Autodesk Inventor part; units mm, degrees
(part 2 of 4)
sketch "Sketch7" plane through (0, 0, 0.5) normal (0, 0, 1) x (1, 0, 0)
  line L0 (29.16, -27.5) -> (28.16, -27.5)
  line L1 (28.16, -27.5) -> (28.16, -25)
  line L2 (28.16, -25) -> (29.16, -25)
  line L3 (29.16, -25) -> (29.16, -27.5)
  line L4 (24.08, -27.5) -> (23.08, -27.5)
  line L5 (23.08, -27.5) -> (23.08, -25)
  line L6 (23.08, -25) -> (24.08, -25)
  line L7 (24.08, -25) -> (24.08, -27.5)
  line L8 (19, -25) -> (19, -27.5)
  line L9 (19, -27.5) -> (18, -27.5)
  line L10 (18, -27.5) -> (18, -25)
  line L11 (18, -25) -> (19, -25)
  line L12 (14.85, -3.9) -> (13.65, -3.9)
  line L13 (13.65, -3.9) -> (13.65, -3.6)
  line L14 (13.65, -3.6) -> (14.85, -3.6)
  line L15 (14.85, -3.6) -> (14.85, -3.9)
  line L16 (14.85, -3.4) -> (13.65, -3.4)
  line L17 (13.65, -3.4) -> (13.65, -3.1)
  line L18 (13.65, -3.1) -> (14.85, -3.1)
  line L19 (14.85, -3.1) -> (14.85, -3.4)
  line L20 (14.85, -2.9) -> (13.65, -2.9)
  line L21 (13.65, -2.9) -> (13.65, -2.6)
  line L22 (13.65, -2.6) -> (14.85, -2.6)
  line L23 (14.85, -2.6) -> (14.85, -2.9)
  line L24 (14.85, -2.4) -> (13.65, -2.4)
  line L25 (13.65, -2.4) -> (13.65, -2.1)
  line L26 (13.65, -2.1) -> (14.85, -2.1)
  line L27 (14.85, -2.1) -> (14.85, -2.4)
  line L28 (14.85, -1.9) -> (13.65, -1.9)
  line L29 (13.65, -1.9) -> (13.65, -1.6)
  line L30 (13.65, -1.6) -> (14.85, -1.6)
  line L31 (14.85, -1.6) -> (14.85, -1.9)
  line L32 (14.85, -1.4) -> (13.65, -1.4)
  line L33 (13.65, -1.4) -> (13.65, -1.1)
  line L34 (13.65, -1.1) -> (14.85, -1.1)
  line L35 (14.85, -1.1) -> (14.85, -1.4)
  line L36 (14.85, -0.9) -> (13.65, -0.9)
  line L37 (13.65, -0.9) -> (13.65, -0.6)
  line L38 (13.65, -0.6) -> (14.85, -0.6)
  line L39 (14.85, -0.6) -> (14.85, -0.9)
  line L40 (14.85, -0.4) -> (13.65, -0.4)
  line L41 (13.65, -0.4) -> (13.65, -0.1)
  line L42 (13.65, -0.1) -> (14.85, -0.1)
  line L43 (14.85, -0.1) -> (14.85, -0.4)
  line L44 (14.85, 0.1) -> (13.65, 0.1)
  line L45 (13.65, 0.1) -> (13.65, 0.4)
  line L46 (13.65, 0.4) -> (14.85, 0.4)
  line L47 (14.85, 0.4) -> (14.85, 0.1)
  line L48 (14.85, 0.6) -> (13.65, 0.6)
  line L49 (13.65, 0.6) -> (13.65, 0.9)
  line L50 (13.65, 0.9) -> (14.85, 0.9)
  line L51 (14.85, 0.9) -> (14.85, 0.6)
  line L52 (14.85, 1.1) -> (13.65, 1.1)
  line L53 (13.65, 1.1) -> (13.65, 1.4)
  line L54 (13.65, 1.4) -> (14.85, 1.4)
  line L55 (14.85, 1.4) -> (14.85, 1.1)
  line L56 (14.85, 1.6) -> (13.65, 1.6)
  line L57 (13.65, 1.6) -> (13.65, 1.9)
  line L58 (13.65, 1.9) -> (14.85, 1.9)
  line L59 (14.85, 1.9) -> (14.85, 1.6)
  line L60 (14.85, 2.1) -> (13.65, 2.1)
  line L61 (13.65, 2.1) -> (13.65, 2.4)
  line L62 (13.65, 2.4) -> (14.85, 2.4)
  line L63 (14.85, 2.4) -> (14.85, 2.1)
  line L64 (14.85, 2.6) -> (13.65, 2.6)
  line L65 (13.65, 2.6) -> (13.65, 2.9)
  line L66 (13.65, 2.9) -> (14.85, 2.9)
  line L67 (14.85, 2.9) -> (14.85, 2.6)
  line L68 (14.85, 3.1) -> (13.65, 3.1)
  line L69 (13.65, 3.1) -> (13.65, 3.4)
  line L70 (13.65, 3.4) -> (14.85, 3.4)
  line L71 (14.85, 3.4) -> (14.85, 3.1)
  line L72 (26.35, 3.9) -> (26.35, 3.6)
  line L73 (26.35, 3.6) -> (25.15, 3.6)
  line L74 (25.15, 3.6) -> (25.15, 3.9)
  line L75 (25.15, 3.9) -> (26.35, 3.9)
  line L76 (23.9, 6.35) -> (23.9, 5.15)
  line L77 (23.9, 5.15) -> (23.6, 5.15)
  line L78 (23.6, 5.15) -> (23.6, 6.35)
  line L79 (23.6, 6.35) -> (23.9, 6.35)
  line L80 (23.4, 6.35) -> (23.4, 5.15)
  line L81 (23.4, 5.15) -> (23.1, 5.15)
  line L82 (23.1, 5.15) -> (23.1, 6.35)
  line L83 (23.1, 6.35) -> (23.4, 6.35)
  line L84 (22.9, 6.35) -> (22.9, 5.15)
  line L85 (22.9, 5.15) -> (22.6, 5.15)
  line L86 (22.6, 5.15) -> (22.6, 6.35)
  line L87 (22.6, 6.35) -> (22.9, 6.35)
  line L88 (22.4, 6.35) -> (22.4, 5.15)
  line L89 (22.4, 5.15) -> (22.1, 5.15)
  line L90 (22.1, 5.15) -> (22.1, 6.35)
  line L91 (22.1, 6.35) -> (22.4, 6.35)
  line L92 (21.9, 6.35) -> (21.9, 5.15)
  line L93 (21.9, 5.15) -> (21.6, 5.15)
  line L94 (21.6, 5.15) -> (21.6, 6.35)
  line L95 (21.6, 6.35) -> (21.9, 6.35)
  line L96 (21.4, 6.35) -> (21.4, 5.15)
  line L97 (21.4, 5.15) -> (21.1, 5.15)
  line L98 (21.1, 5.15) -> (21.1, 6.35)
  line L99 (21.1, 6.35) -> (21.4, 6.35)
  line L100 (20.9, 6.35) -> (20.9, 5.15)
  line L101 (20.9, 5.15) -> (20.6, 5.15)
  line L102 (20.6, 5.15) -> (20.6, 6.35)
  line L103 (20.6, 6.35) -> (20.9, 6.35)
  line L104 (20.4, 6.35) -> (20.4, 5.15)
  line L105 (20.4, 5.15) -> (20.1, 5.15)
  line L106 (20.1, 5.15) -> (20.1, 6.35)
  line L107 (20.1, 6.35) -> (20.4, 6.35)
  line L108 (19.9, 6.35) -> (19.9, 5.15)
  line L109 (19.9, 5.15) -> (19.6, 5.15)
  line L110 (19.6, 5.15) -> (19.6, 6.35)
  line L111 (19.6, 6.35) -> (19.9, 6.35)
  line L112 (19.4, 6.35) -> (19.4, 5.15)
  line L113 (19.4, 5.15) -> (19.1, 5.15)
  line L114 (19.1, 5.15) -> (19.1, 6.35)
  line L115 (19.1, 6.35) -> (19.4, 6.35)
  line L116 (18.9, 6.35) -> (18.9, 5.15)
  line L117 (18.9, 5.15) -> (18.6, 5.15)
  line L118 (18.6, 5.15) -> (18.6, 6.35)
  line L119 (18.6, 6.35) -> (18.9, 6.35)
  line L120 (18.4, 6.35) -> (18.4, 5.15)
  line L121 (18.4, 5.15) -> (18.1, 5.15)
  line L122 (18.1, 5.15) -> (18.1, 6.35)
  line L123 (18.1, 6.35) -> (18.4, 6.35)
  line L124 (17.9, 6.35) -> (17.9, 5.15)
  line L125 (17.9, 5.15) -> (17.6, 5.15)
  line L126 (17.6, 5.15) -> (17.6, 6.35)
  line L127 (17.6, 6.35) -> (17.9, 6.35)
  line L128 (17.4, 6.35) -> (17.4, 5.15)
  line L129 (17.4, 5.15) -> (17.1, 5.15)
  line L130 (17.1, 5.15) -> (17.1, 6.35)
  line L131 (17.1, 6.35) -> (17.4, 6.35)
  line L132 (16.9, 6.35) -> (16.9, 5.15)
  line L133 (16.9, 5.15) -> (16.6, 5.15)
  line L134 (16.6, 5.15) -> (16.6, 6.35)
  line L135 (16.6, 6.35) -> (16.9, 6.35)
  line L136 (16.4, 6.35) -> (16.4, 5.15)
  line L137 (16.4, 5.15) -> (16.1, 5.15)
  line L138 (16.1, 5.15) -> (16.1, 6.35)
  line L139 (16.1, 6.35) -> (16.4, 6.35)
  line L140 (16.4, -5.15) -> (16.4, -6.35)
  line L141 (16.4, -6.35) -> (16.1, -6.35)
  line L142 (16.1, -6.35) -> (16.1, -5.15)
  line L143 (16.1, -5.15) -> (16.4, -5.15)
  line L144 (16.9, -5.15) -> (16.9, -6.35)
  line L145 (16.9, -6.35) -> (16.6, -6.35)
  line L146 (16.6, -6.35) -> (16.6, -5.15)
  line L147 (16.6, -5.15) -> (16.9, -5.15)
  line L148 (17.4, -5.15) -> (17.4, -6.35)
  line L149 (17.4, -6.35) -> (17.1, -6.35)
  line L150 (17.1, -6.35) -> (17.1, -5.15)
  line L151 (17.1, -5.15) -> (17.4, -5.15)
  line L152 (17.9, -5.15) -> (17.9, -6.35)
  line L153 (17.9, -6.35) -> (17.6, -6.35)
  line L154 (17.6, -6.35) -> (17.6, -5.15)
  line L155 (17.6, -5.15) -> (17.9, -5.15)
  line L156 (18.4, -5.15) -> (18.4, -6.35)
  line L157 (18.4, -6.35) -> (18.1, -6.35)
  line L158 (18.1, -6.35) -> (18.1, -5.15)
  line L159 (18.1, -5.15) -> (18.4, -5.15)
  line L160 (18.9, -5.15) -> (18.9, -6.35)
  line L161 (18.9, -6.35) -> (18.6, -6.35)
  line L162 (18.6, -6.35) -> (18.6, -5.15)
  line L163 (18.6, -5.15) -> (18.9, -5.15)
  line L164 (19.4, -5.15) -> (19.4, -6.35)
  line L165 (19.4, -6.35) -> (19.1, -6.35)
  line L166 (19.1, -6.35) -> (19.1, -5.15)
  line L167 (19.1, -5.15) -> (19.4, -5.15)
  line L168 (19.9, -5.15) -> (19.9, -6.35)
  line L169 (19.9, -6.35) -> (19.6, -6.35)
  line L170 (19.6, -6.35) -> (19.6, -5.15)
  line L171 (19.6, -5.15) -> (19.9, -5.15)
  line L172 (20.4, -5.15) -> (20.4, -6.35)
  line L173 (20.4, -6.35) -> (20.1, -6.35)
  line L174 (20.1, -6.35) -> (20.1, -5.15)
  line L175 (20.1, -5.15) -> (20.4, -5.15)
  line L176 (20.9, -5.15) -> (20.9, -6.35)
  line L177 (20.9, -6.35) -> (20.6, -6.35)
  line L178 (20.6, -6.35) -> (20.6, -5.15)
  line L179 (20.6, -5.15) -> (20.9, -5.15)
  line L180 (21.4, -5.15) -> (21.4, -6.35)
  line L181 (21.4, -6.35) -> (21.1, -6.35)
  line L182 (21.1, -6.35) -> (21.1, -5.15)
  line L183 (21.1, -5.15) -> (21.4, -5.15)
  line L184 (21.9, -5.15) -> (21.9, -6.35)
  line L185 (21.9, -6.35) -> (21.6, -6.35)
  line L186 (21.6, -6.35) -> (21.6, -5.15)
  line L187 (21.6, -5.15) -> (21.9, -5.15)
  line L188 (22.4, -5.15) -> (22.4, -6.35)
  line L189 (22.4, -6.35) -> (22.1, -6.35)
  line L190 (22.1, -6.35) -> (22.1, -5.15)
  line L191 (22.1, -5.15) -> (22.4, -5.15)
  line L192 (22.9, -5.15) -> (22.9, -6.35)
  line L193 (22.9, -6.35) -> (22.6, -6.35)
  line L194 (22.6, -6.35) -> (22.6, -5.15)
  line L195 (22.6, -5.15) -> (22.9, -5.15)
  line L196 (23.4, -5.15) -> (23.4, -6.35)
  line L197 (23.4, -6.35) -> (23.1, -6.35)
  line L198 (23.1, -6.35) -> (23.1, -5.15)
  line L199 (23.1, -5.15) -> (23.4, -5.15)
  line L200 (23.9, -5.15) -> (23.9, -6.35)
  line L201 (23.9, -6.35) -> (23.6, -6.35)
  line L202 (23.6, -6.35) -> (23.6, -5.15)
  line L203 (23.6, -5.15) -> (23.9, -5.15)
  line L204 (14.85, 3.9) -> (14.85, 3.6)
  line L205 (14.85, 3.6) -> (13.65, 3.6)
  line L206 (13.65, 3.6) -> (13.65, 3.9)
  line L207 (13.65, 3.9) -> (14.85, 3.9)
  line L208 (26.35, 3.4) -> (26.35, 3.1)
  line L209 (26.35, 3.1) -> (25.15, 3.1)
  line L210 (25.15, 3.1) -> (25.15, 3.4)
  line L211 (25.15, 3.4) -> (26.35, 3.4)
  line L212 (26.35, 2.9) -> (26.35, 2.6)
  line L213 (26.35, 2.6) -> (25.15, 2.6)
  line L214 (25.15, 2.6) -> (25.15, 2.9)
  line L215 (25.15, 2.9) -> (26.35, 2.9)
  line L216 (26.35, 2.4) -> (26.35, 2.1)
  line L217 (26.35, 2.1) -> (25.15, 2.1)
  line L218 (25.15, 2.1) -> (25.15, 2.4)
  line L219 (25.15, 2.4) -> (26.35, 2.4)
  line L220 (26.35, 1.9) -> (26.35, 1.6)
  line L221 (26.35, 1.6) -> (25.15, 1.6)
  line L222 (25.15, 1.6) -> (25.15, 1.9)
  line L223 (25.15, 1.9) -> (26.35, 1.9)
  line L224 (26.35, 1.4) -> (26.35, 1.1)
  line L225 (26.35, 1.1) -> (25.15, 1.1)
  line L226 (25.15, 1.1) -> (25.15, 1.4)
  line L227 (25.15, 1.4) -> (26.35, 1.4)
  line L228 (26.35, 0.9) -> (26.35, 0.6)
  line L229 (26.35, 0.6) -> (25.15, 0.6)
  line L230 (25.15, 0.6) -> (25.15, 0.9)
  line L231 (25.15, 0.9) -> (26.35, 0.9)
  line L232 (26.35, 0.4) -> (26.35, 0.1)
  line L233 (26.35, 0.1) -> (25.15, 0.1)
  line L234 (25.15, 0.1) -> (25.15, 0.4)
  line L235 (25.15, 0.4) -> (26.35, 0.4)
  line L236 (26.35, -0.1) -> (26.35, -0.4)
  line L237 (26.35, -0.4) -> (25.15, -0.4)
  line L238 (25.15, -0.4) -> (25.15, -0.1)
  line L239 (25.15, -0.1) -> (26.35, -0.1)
  line L240 (26.35, -0.6) -> (26.35, -0.9)
  line L241 (26.35, -0.9) -> (25.15, -0.9)
  line L242 (25.15, -0.9) -> (25.15, -0.6)
  line L243 (25.15, -0.6) -> (26.35, -0.6)
  line L244 (26.35, -1.1) -> (26.35, -1.4)
  line L245 (26.35, -1.4) -> (25.15, -1.4)
  line L246 (25.15, -1.4) -> (25.15, -1.1)
  line L247 (25.15, -1.1) -> (26.35, -1.1)
  line L248 (26.35, -1.6) -> (26.35, -1.9)
  line L249 (26.35, -1.9) -> (25.15, -1.9)
  line L250 (25.15, -1.9) -> (25.15, -1.6)
  line L251 (25.15, -1.6) -> (26.35, -1.6)
  line L252 (26.35, -2.1) -> (26.35, -2.4)
  line L253 (26.35, -2.4) -> (25.15, -2.4)
  line L254 (25.15, -2.4) -> (25.15, -2.1)
  line L255 (25.15, -2.1) -> (26.35, -2.1)
  line L256 (26.35, -2.6) -> (26.35, -2.9)
  line L257 (26.35, -2.9) -> (25.15, -2.9)
  line L258 (25.15, -2.9) -> (25.15, -2.6)
  line L259 (25.15, -2.6) -> (26.35, -2.6)
  line L260 (26.35, -3.1) -> (26.35, -3.4)
  line L261 (26.35, -3.4) -> (25.15, -3.4)
  line L262 (25.15, -3.4) -> (25.15, -3.1)
  line L263 (25.15, -3.1) -> (26.35, -3.1)
  line L264 (26.35, -3.6) -> (26.35, -3.9)
  line L265 (26.35, -3.9) -> (25.15, -3.9)
  line L266 (25.15, -3.9) -> (25.15, -3.6)
  line L267 (25.15, -3.6) -> (26.35, -3.6)
  line L268 (21.54, -27.5) -> (20.54, -27.5)
  line L269 (20.54, -27.5) -> (20.54, -25)
  line L270 (20.54, -25) -> (21.54, -25)
  line L271 (21.54, -25) -> (21.54, -27.5)
  line L272 (26.62, -27.5) -> (25.62, -27.5)
  line L273 (25.62, -27.5) -> (25.62, -25)
  line L274 (25.62, -25) -> (26.62, -25)
  line L275 (26.62, -25) -> (26.62, -27.5)
  line L276 (31.7, -27.5) -> (30.7, -27.5)
  line L277 (30.7, -27.5) -> (30.7, -25)
  line L278 (30.7, -25) -> (31.7, -25)
  line L279 (31.7, -25) -> (31.7, -27.5)
  line L280 (79.1, -4.35) -> (79.1, -3.35)
  line L281 (79.1, -3.35) -> (82.4, -3.35)
  line L282 (82.4, -3.35) -> (82.4, -5.9)
  line L283 (82.4, -5.9) -> (81.4, -5.9)
  line L284 (81.4, -5.9) -> (81.4, -4.35)
  line L285 (81.4, -4.35) -> (79.1, -4.35)
  line L286 (37.6, -34.65) -> (37.6, -32.1)
  line L287 (37.6, -32.1) -> (38.6, -32.1)
  line L288 (38.6, -32.1) -> (38.6, -33.65)
  line L289 (38.6, -33.65) -> (40.9, -33.65)
  line L290 (40.9, -33.65) -> (40.9, -34.65)
  line L291 (40.9, -34.65) -> (37.6, -34.65)
  line L292 (70.9, -3.35) -> (70.9, -4.35)
  line L293 (70.9, -4.35) -> (67.1, -4.35)
  line L294 (67.1, -4.35) -> (67.1, -3.35)
  line L295 (67.1, -3.35) -> (70.9, -3.35)
  line L296 (73.1, -33.65) -> (76.9, -33.65)
  line L297 (76.9, -33.65) -> (76.9, -34.65)
  line L298 (76.9, -34.65) -> (73.1, -34.65)
  line L299 (73.1, -34.65) -> (73.1, -33.65)
  line L300 (81.4, -20.1) -> (82.4, -20.1)
  line L301 (82.4, -20.1) -> (82.4, -23.9)
  line L302 (82.4, -23.9) -> (81.4, -23.9)
  line L303 (81.4, -23.9) -> (81.4, -20.1)
  line L304 (46.9, -3.35) -> (46.9, -4.35)
  line L305 (46.9, -4.35) -> (43.1, -4.35)
  line L306 (43.1, -4.35) -> (43.1, -3.35)
  line L307 (43.1, -3.35) -> (46.9, -3.35)
  line L308 (58.9, -3.35) -> (58.9, -4.35)
  line L309 (58.9, -4.35) -> (55.1, -4.35)
  line L310 (55.1, -4.35) -> (55.1, -3.35)
  line L311 (55.1, -3.35) -> (58.9, -3.35)
  line L312 (61.1, -33.65) -> (64.9, -33.65)
  line L313 (64.9, -33.65) -> (64.9, -34.65)
  line L314 (64.9, -34.65) -> (61.1, -34.65)
  line L315 (61.1, -34.65) -> (61.1, -33.65)
  line L316 (49.1, -33.65) -> (52.9, -33.65)
  line L317 (52.9, -33.65) -> (52.9, -34.65)
  line L318 (52.9, -34.65) -> (49.1, -34.65)
  line L319 (49.1, -34.65) -> (49.1, -33.65)
  line L320 (81.4, -26.1) -> (82.4, -26.1)
  line L321 (82.4, -26.1) -> (82.4, -29.9)
  line L322 (82.4, -29.9) -> (81.4, -29.9)
  line L323 (81.4, -29.9) -> (81.4, -26.1)
  line L324 (81.4, -8.1) -> (82.4, -8.1)
  line L325 (82.4, -8.1) -> (82.4, -11.9)
  line L326 (82.4, -11.9) -> (81.4, -11.9)
  line L327 (81.4, -11.9) -> (81.4, -8.1)
  line L328 (37.6, -17.9) -> (37.6, -14.1)
  line L329 (37.6, -14.1) -> (38.6, -14.1)
  line L330 (38.6, -14.1) -> (38.6, -17.9)
  line L331 (38.6, -17.9) -> (37.6, -17.9)
  line L332 (86.1, -25.4) -> (86.1, -26.75)
  line L333 (86.1, -26.75) -> (83.9, -26.75)
  line L334 (83.9, -26.75) -> (83.9, -25.4)
  line L335 (83.9, -25.4) -> (83.4, -25.4)
  line L336 (83.4, -25.4) -> (83.4, -24.6)
  line L337 (83.4, -24.6) -> (83.9, -24.6)
  line L338 (83.9, -24.6) -> (83.9, -23.25)
  line L339 (83.9, -23.25) -> (86.1, -23.25)
  line L340 (86.1, -23.25) -> (86.1, -24.6)
  line L341 (86.1, -24.6) -> (86.6, -24.6)
  line L342 (86.6, -24.6) -> (86.6, -25.4)
  line L343 (86.6, -25.4) -> (86.1, -25.4)
  line L344 (37.6, -29.9) -> (37.6, -26.1)
  line L345 (37.6, -26.1) -> (38.6, -26.1)
  line L346 (38.6, -26.1) -> (38.6, -29.9)
  line L347 (38.6, -29.9) -> (37.6, -29.9)
  line L348 (37.6, -11.9) -> (37.6, -8.1)
  line L349 (37.6, -8.1) -> (38.6, -8.1)
  line L350 (38.6, -8.1) -> (38.6, -11.9)
  line L351 (38.6, -11.9) -> (37.6, -11.9)
  line L352 (81.4, -14.1) -> (82.4, -14.1)
  line L353 (82.4, -14.1) -> (82.4, -17.9)
  line L354 (82.4, -17.9) -> (81.4, -17.9)
  line L355 (81.4, -17.9) -> (81.4, -14.1)
  line L356 (43.1, -33.65) -> (46.9, -33.65)
  line L357 (46.9, -33.65) -> (46.9, -34.65)
  line L358 (46.9, -34.65) -> (43.1, -34.65)
  line L359 (43.1, -34.65) -> (43.1, -33.65)
  line L360 (55.1, -33.65) -> (58.9, -33.65)
  line L361 (58.9, -33.65) -> (58.9, -34.65)
  line L362 (58.9, -34.65) -> (55.1, -34.65)
  line L363 (55.1, -34.65) -> (55.1, -33.65)
  line L364 (64.9, -3.35) -> (64.9, -4.35)
  line L365 (64.9, -4.35) -> (61.1, -4.35)
  line L366 (61.1, -4.35) -> (61.1, -3.35)
  line L367 (61.1, -3.35) -> (64.9, -3.35)
  line L368 (52.9, -3.35) -> (52.9, -4.35)
  line L369 (52.9, -4.35) -> (49.1, -4.35)
  line L370 (49.1, -4.35) -> (49.1, -3.35)
  line L371 (49.1, -3.35) -> (52.9, -3.35)
  line L372 (37.6, -23.9) -> (37.6, -20.1)
  line L373 (37.6, -20.1) -> (38.6, -20.1)
  line L374 (38.6, -20.1) -> (38.6, -23.9)
  line L375 (38.6, -23.9) -> (37.6, -23.9)
  line L376 (70.9, -33.65) -> (70.9, -34.65)
  line L377 (70.9, -34.65) -> (67.1, -34.65)
  line L378 (67.1, -34.65) -> (67.1, -33.65)
  line L379 (67.1, -33.65) -> (70.9, -33.65)
  line L380 (76.9, -3.35) -> (76.9, -4.35)
  line L381 (76.9, -4.35) -> (73.1, -4.35)
  line L382 (73.1, -4.35) -> (73.1, -3.35)
  line L383 (73.1, -3.35) -> (76.9, -3.35)
  line L384 (37.6, -3.35) -> (40.9, -3.35)
  line L385 (40.9, -3.35) -> (40.9, -4.35)
  line L386 (40.9, -4.35) -> (38.6, -4.35)
  line L387 (38.6, -4.35) -> (38.6, -5.9)
  line L388 (38.6, -5.9) -> (37.6, -5.9)
  line L389 (37.6, -5.9) -> (37.6, -3.35)
  line L390 (79.1, -33.65) -> (81.4, -33.65)
  line L391 (81.4, -33.65) -> (81.4, -32.1)
  line L392 (81.4, -32.1) -> (82.4, -32.1)
  line L393 (82.4, -32.1) -> (82.4, -34.65)
  line L394 (82.4, -34.65) -> (79.1, -34.65)
  line L395 (79.1, -34.65) -> (79.1, -33.65)
  line L396 (79.1, 35.65) -> (79.1, 36.65)
  line L397 (79.1, 36.65) -> (82.4, 36.65)
  line L398 (82.4, 36.65) -> (82.4, 34.1)
  line L399 (82.4, 34.1) -> (81.4, 34.1)
  line L400 (81.4, 34.1) -> (81.4, 35.65)
  line L401 (81.4, 35.65) -> (79.1, 35.65)
  line L402 (37.6, 5.35) -> (37.6, 7.9)
  line L403 (37.6, 7.9) -> (38.6, 7.9)
  line L404 (38.6, 7.9) -> (38.6, 6.35)
  line L405 (38.6, 6.35) -> (40.9, 6.35)
  line L406 (40.9, 6.35) -> (40.9, 5.35)
  line L407 (40.9, 5.35) -> (37.6, 5.35)
  line L408 (70.9, 36.65) -> (70.9, 35.65)
  line L409 (70.9, 35.65) -> (67.1, 35.65)
  line L410 (67.1, 35.65) -> (67.1, 36.65)
  line L411 (67.1, 36.65) -> (70.9, 36.65)
  line L412 (73.1, 6.35) -> (76.9, 6.35)
  line L413 (76.9, 6.35) -> (76.9, 5.35)
  line L414 (76.9, 5.35) -> (73.1, 5.35)
  line L415 (73.1, 5.35) -> (73.1, 6.35)
  line L416 (81.4, 19.9) -> (82.4, 19.9)
  line L417 (82.4, 19.9) -> (82.4, 16.1)
  line L418 (82.4, 16.1) -> (81.4, 16.1)
  line L419 (81.4, 16.1) -> (81.4, 19.9)
  line L420 (46.9, 36.65) -> (46.9, 35.65)
  line L421 (46.9, 35.65) -> (43.1, 35.65)
  line L422 (43.1, 35.65) -> (43.1, 36.65)
  line L423 (43.1, 36.65) -> (46.9, 36.65)
  line L424 (58.9, 36.65) -> (58.9, 35.65)
  line L425 (58.9, 35.65) -> (55.1, 35.65)
  line L426 (55.1, 35.65) -> (55.1, 36.65)
  line L427 (55.1, 36.65) -> (58.9, 36.65)
  line L428 (61.1, 6.35) -> (64.9, 6.35)
  line L429 (64.9, 6.35) -> (64.9, 5.35)
  line L430 (64.9, 5.35) -> (61.1, 5.35)
  line L431 (61.1, 5.35) -> (61.1, 6.35)
  line L432 (49.1, 6.35) -> (52.9, 6.35)
  line L433 (52.9, 6.35) -> (52.9, 5.35)
  line L434 (52.9, 5.35) -> (49.1, 5.35)
  line L435 (49.1, 5.35) -> (49.1, 6.35)
  line L436 (81.4, 13.9) -> (82.4, 13.9)
  line L437 (82.4, 13.9) -> (82.4, 10.1)
  line L438 (82.4, 10.1) -> (81.4, 10.1)
  line L439 (81.4, 10.1) -> (81.4, 13.9)
  line L440 (81.4, 31.9) -> (82.4, 31.9)
  line L441 (82.4, 31.9) -> (82.4, 28.1)
  line L442 (82.4, 28.1) -> (81.4, 28.1)
  line L443 (81.4, 28.1) -> (81.4, 31.9)
  line L444 (37.6, 22.1) -> (37.6, 25.9)
  line L445 (37.6, 25.9) -> (38.6, 25.9)
  line L446 (38.6, 25.9) -> (38.6, 22.1)
  line L447 (38.6, 22.1) -> (37.6, 22.1)
  line L448 (86.1, 14.6) -> (86.1, 13.25)
  line L449 (86.1, 13.25) -> (83.9, 13.25)
  line L450 (83.9, 13.25) -> (83.9, 14.6)
  line L451 (83.9, 14.6) -> (83.4, 14.6)
  line L452 (83.4, 14.6) -> (83.4, 15.4)
  line L453 (83.4, 15.4) -> (83.9, 15.4)
  line L454 (83.9, 15.4) -> (83.9, 16.75)
  line L455 (83.9, 16.75) -> (86.1, 16.75)
  line L456 (86.1, 16.75) -> (86.1, 15.4)
  line L457 (86.1, 15.4) -> (86.6, 15.4)
  line L458 (86.6, 15.4) -> (86.6, 14.6)
  line L459 (86.6, 14.6) -> (86.1, 14.6)
  line L460 (37.6, 10.1) -> (37.6, 13.9)
  line L461 (37.6, 13.9) -> (38.6, 13.9)
  line L462 (38.6, 13.9) -> (38.6, 10.1)
  line L463 (38.6, 10.1) -> (37.6, 10.1)
  line L464 (37.6, 28.1) -> (37.6, 31.9)
  line L465 (37.6, 31.9) -> (38.6, 31.9)
  line L466 (38.6, 31.9) -> (38.6, 28.1)
  line L467 (38.6, 28.1) -> (37.6, 28.1)
  line L468 (81.4, 25.9) -> (82.4, 25.9)
  line L469 (82.4, 25.9) -> (82.4, 22.1)
  line L470 (82.4, 22.1) -> (81.4, 22.1)
  line L471 (81.4, 22.1) -> (81.4, 25.9)
  line L472 (43.1, 6.35) -> (46.9, 6.35)
  line L473 (46.9, 6.35) -> (46.9, 5.35)
  line L474 (46.9, 5.35) -> (43.1, 5.35)
  line L475 (43.1, 5.35) -> (43.1, 6.35)
  line L476 (55.1, 6.35) -> (58.9, 6.35)
  line L477 (58.9, 6.35) -> (58.9, 5.35)
  line L478 (58.9, 5.35) -> (55.1, 5.35)
  line L479 (55.1, 5.35) -> (55.1, 6.35)
  line L480 (64.9, 36.65) -> (64.9, 35.65)
  line L481 (64.9, 35.65) -> (61.1, 35.65)
  line L482 (61.1, 35.65) -> (61.1, 36.65)
  line L483 (61.1, 36.65) -> (64.9, 36.65)
  line L484 (52.9, 36.65) -> (52.9, 35.65)
  line L485 (52.9, 35.65) -> (49.1, 35.65)
  line L486 (49.1, 35.65) -> (49.1, 36.65)
  line L487 (49.1, 36.65) -> (52.9, 36.65)
  line L488 (37.6, 16.1) -> (37.6, 19.9)
  line L489 (37.6, 19.9) -> (38.6, 19.9)
  line L490 (38.6, 19.9) -> (38.6, 16.1)
  line L491 (38.6, 16.1) -> (37.6, 16.1)
  line L492 (70.9, 6.35) -> (70.9, 5.35)
  line L493 (70.9, 5.35) -> (67.1, 5.35)
  line L494 (67.1, 5.35) -> (67.1, 6.35)
  line L495 (67.1, 6.35) -> (70.9, 6.35)
  line L496 (76.9, 36.65) -> (76.9, 35.65)
  line L497 (76.9, 35.65) -> (73.1, 35.65)
  line L498 (73.1, 35.65) -> (73.1, 36.65)
  line L499 (73.1, 36.65) -> (76.9, 36.65)
  line L500 (37.6, 36.65) -> (40.9, 36.65)
  line L501 (40.9, 36.65) -> (40.9, 35.65)
  line L502 (40.9, 35.65) -> (38.6, 35.65)
  line L503 (38.6, 35.65) -> (38.6, 34.1)
  line L504 (38.6, 34.1) -> (37.6, 34.1)
  line L505 (37.6, 34.1) -> (37.6, 36.65)
  line L506 (79.1, 6.35) -> (81.4, 6.35)
  line L507 (81.4, 6.35) -> (81.4, 7.9)
  line L508 (81.4, 7.9) -> (82.4, 7.9)
  line L509 (82.4, 7.9) -> (82.4, 5.35)
  line L510 (82.4, 5.35) -> (79.1, 5.35)
  line L511 (79.1, 5.35) -> (79.1, 6.35)
  line L512 (0, 18.95) -> (3.5, 18.95)
  arc A0 (3.5, 17.95) -> (3.5, 18.95) centre (3.5, 18.45) ccw
  line L513 (3.5, 17.95) -> (0, 17.95)
  line L514 (0, 17.95) -> (0, -33.8)
  line L515 (0, -33.8) -> (12.5, -33.8)
  line L516 (12.5, -33.8) -> (12.5, -45.4)
  line L517 (12.5, -45.4) -> (91.4, -45.4)
  line L518 (91.4, -45.4) -> (91.4, 45.4)
  line L519 (91.4, 45.4) -> (12.5, 45.4)
  line L520 (12.5, 45.4) -> (12.5, 33.8)
  line L521 (12.5, 33.8) -> (0, 33.8)
  line L522 (0, 33.8) -> (0, 18.95)
  circle A1 centre (6, -31.8) radius 0.9
  circle A2 centre (6, 31.8) radius 0.9
  line L523 (0.25, 31.875) -> (2.8, 31.875)
  line L524 (2.8, 31.875) -> (2.8, 31.425)
  line L525 (2.8, 31.425) -> (0.25, 31.425)
  line L526 (0.25, 31.425) -> (0.25, 31.875)
  line L527 (0.25, 16.275) -> (2.8, 16.275)
  line L528 (2.8, 16.275) -> (2.8, 15.825)
  line L529 (2.8, 15.825) -> (0.25, 15.825)
  line L530 (0.25, 15.825) -> (0.25, 16.275)
  line L531 (2.8, 31.275) -> (2.8, 30.825)
  line L532 (0.25, 30.825) -> (0.25, 31.275)
  line L533 (2.8, 30.825) -> (0.25, 30.825)
  line L534 (0.25, 31.275) -> (2.8, 31.275)
  line L535 (2.8, 30.675) -> (2.8, 30.225)
  line L536 (0.25, 30.225) -> (0.25, 30.675)
  line L537 (2.8, 30.225) -> (0.25, 30.225)
  line L538 (0.25, 30.675) -> (2.8, 30.675)
  line L539 (2.8, 30.075) -> (2.8, 29.625)
  line L540 (0.25, 29.625) -> (0.25, 30.075)
  line L541 (2.8, 29.625) -> (0.25, 29.625)
  line L542 (0.25, 30.075) -> (2.8, 30.075)
  line L543 (2.8, 29.475) -> (2.8, 29.025)
  line L544 (0.25, 29.025) -> (0.25, 29.475)
  line L545 (2.8, 29.025) -> (0.25, 29.025)
  line L546 (0.25, 29.475) -> (2.8, 29.475)
  line L547 (2.8, 28.875) -> (2.8, 28.425)
  line L548 (0.25, 28.425) -> (0.25, 28.875)
  line L549 (2.8, 28.425) -> (0.25, 28.425)
  line L550 (0.25, 28.875) -> (2.8, 28.875)
  line L551 (2.8, 28.275) -> (2.8, 27.825)
  line L552 (0.25, 27.825) -> (0.25, 28.275)
  line L553 (2.8, 27.825) -> (0.25, 27.825)
  line L554 (0.25, 28.275) -> (2.8, 28.275)
  line L555 (2.8, 27.675) -> (2.8, 27.225)
  line L556 (0.25, 27.225) -> (0.25, 27.675)
  line L557 (2.8, 27.225) -> (0.25, 27.225)
  line L558 (0.25, 27.675) -> (2.8, 27.675)
  line L559 (2.8, 27.075) -> (2.8, 26.625)
  line L560 (0.25, 26.625) -> (0.25, 27.075)
  line L561 (2.8, 26.625) -> (0.25, 26.625)
  line L562 (0.25, 27.075) -> (2.8, 27.075)
  line L563 (2.8, 26.475) -> (2.8, 26.025)
  line L564 (0.25, 26.025) -> (0.25, 26.475)
  line L565 (2.8, 26.025) -> (0.25, 26.025)
  line L566 (0.25, 26.475) -> (2.8, 26.475)
  line L567 (2.8, 25.875) -> (2.8, 25.425)
  line L568 (0.25, 25.425) -> (0.25, 25.875)
  line L569 (2.8, 25.425) -> (0.25, 25.425)
  line L570 (0.25, 25.875) -> (2.8, 25.875)
  line L571 (2.8, 25.275) -> (2.8, 24.825)
  line L572 (0.25, 24.825) -> (0.25, 25.275)
  line L573 (2.8, 24.825) -> (0.25, 24.825)
  line L574 (0.25, 25.275) -> (2.8, 25.275)
  line L575 (2.8, 24.675) -> (2.8, 24.225)
  line L576 (0.25, 24.225) -> (0.25, 24.675)
  line L577 (2.8, 24.225) -> (0.25, 24.225)
  line L578 (0.25, 24.675) -> (2.8, 24.675)
  line L579 (2.8, 24.075) -> (2.8, 23.625)
  line L580 (0.25, 23.625) -> (0.25, 24.075)
  line L581 (2.8, 23.625) -> (0.25, 23.625)
  line L582 (0.25, 24.075) -> (2.8, 24.075)
  line L583 (2.8, 23.475) -> (2.8, 23.025)
  line L584 (0.25, 23.025) -> (0.25, 23.475)
  line L585 (2.8, 23.025) -> (0.25, 23.025)
  line L586 (0.25, 23.475) -> (2.8, 23.475)
  line L587 (2.8, 22.875) -> (2.8, 22.425)
  line L588 (0.25, 22.425) -> (0.25, 22.875)
  line L589 (2.8, 22.425) -> (0.25, 22.425)
  line L590 (0.25, 22.875) -> (2.8, 22.875)
  line L591 (2.8, 22.275) -> (2.8, 21.825)
  line L592 (0.25, 21.825) -> (0.25, 22.275)
  line L593 (2.8, 21.825) -> (0.25, 21.825)
  line L594 (0.25, 22.275) -> (2.8, 22.275)
  line L595 (2.8, 21.675) -> (2.8, 21.225)
  line L596 (0.25, 21.225) -> (0.25, 21.675)
  line L597 (2.8, 21.225) -> (0.25, 21.225)
  line L598 (0.25, 21.675) -> (2.8, 21.675)
  line L599 (2.8, 21.075) -> (2.8, 20.625)
  line L600 (0.25, 20.625) -> (0.25, 21.075)
  line L601 (2.8, 20.625) -> (0.25, 20.625)
  line L602 (0.25, 21.075) -> (2.8, 21.075)
  line L603 (2.8, 20.475) -> (2.8, 20.025)
  line L604 (0.25, 20.025) -> (0.25, 20.475)
  line L605 (2.8, 20.025) -> (0.25, 20.025)
  line L606 (0.25, 20.475) -> (2.8, 20.475)
  line L607 (0.25, 15.675) -> (2.8, 15.675)
  line L608 (2.8, 15.675) -> (2.8, 15.225)
  line L609 (2.8, 15.225) -> (0.25, 15.225)
  line L610 (0.25, 15.225) -> (0.25, 15.675)
  line L611 (0.25, 15.075) -> (2.8, 15.075)
  line L612 (2.8, 15.075) -> (2.8, 14.625)
  line L613 (2.8, 14.625) -> (0.25, 14.625)
  line L614 (0.25, 14.625) -> (0.25, 15.075)
  line L615 (0.25, 14.475) -> (2.8, 14.475)
  line L616 (2.8, 14.475) -> (2.8, 14.025)
  line L617 (2.8, 14.025) -> (0.25, 14.025)
  line L618 (0.25, 14.025) -> (0.25, 14.475)
  line L619 (0.25, 13.875) -> (2.8, 13.875)
  line L620 (2.8, 13.875) -> (2.8, 13.425)
  line L621 (2.8, 13.425) -> (0.25, 13.425)
  line L622 (0.25, 13.425) -> (0.25, 13.875)
  line L623 (0.25, 13.275) -> (2.8, 13.275)
  line L624 (2.8, 13.275) -> (2.8, 12.825)
  line L625 (2.8, 12.825) -> (0.25, 12.825)
  line L626 (0.25, 12.825) -> (0.25, 13.275)
  line L627 (0.25, 12.675) -> (2.8, 12.675)
  line L628 (2.8, 12.675) -> (2.8, 12.225)
  line L629 (2.8, 12.225) -> (0.25, 12.225)
  line L630 (0.25, 12.225) -> (0.25, 12.675)
  line L631 (0.25, 12.075) -> (2.8, 12.075)
  line L632 (2.8, 12.075) -> (2.8, 11.625)
  line L633 (2.8, 11.625) -> (0.25, 11.625)
  line L634 (0.25, 11.625) -> (0.25, 12.075)
  line L635 (0.25, 11.475) -> (2.8, 11.475)
  line L636 (2.8, 11.475) -> (2.8, 11.025)
  line L637 (2.8, 11.025) -> (0.25, 11.025)
  line L638 (0.25, 11.025) -> (0.25, 11.475)
  line L639 (0.25, 10.875) -> (2.8, 10.875)
  line L640 (2.8, 10.875) -> (2.8, 10.425)
  line L641 (2.8, 10.425) -> (0.25, 10.425)
  line L642 (0.25, 10.425) -> (0.25, 10.875)
  line L643 (0.25, 10.275) -> (2.8, 10.275)
  line L644 (2.8, 10.275) -> (2.8, 9.825)
  line L645 (2.8, 9.825) -> (0.25, 9.825)
  line L646 (0.25, 9.825) -> (0.25, 10.275)
  line L647 (0.25, 9.675) -> (2.8, 9.675)
  line L648 (2.8, 9.675) -> (2.8, 9.225)
  line L649 (2.8, 9.225) -> (0.25, 9.225)
  line L650 (0.25, 9.225) -> (0.25, 9.675)
  line L651 (0.25, 9.075) -> (2.8, 9.075)
  line L652 (2.8, 9.075) -> (2.8, 8.625)
  line L653 (2.8, 8.625) -> (0.25, 8.625)
  line L654 (0.25, 8.625) -> (0.25, 9.075)
  line L655 (0.25, 8.475) -> (2.8, 8.475)
  line L656 (2.8, 8.475) -> (2.8, 8.025)
  line L657 (2.8, 8.025) -> (0.25, 8.025)
  line L658 (0.25, 8.025) -> (0.25, 8.475)
  line L659 (0.25, 7.875) -> (2.8, 7.875)
  line L660 (2.8, 7.875) -> (2.8, 7.425)
  line L661 (2.8, 7.425) -> (0.25, 7.425)
  line L662 (0.25, 7.425) -> (0.25, 7.875)
  line L663 (0.25, 7.275) -> (2.8, 7.275)
  line L664 (2.8, 7.275) -> (2.8, 6.825)
  line L665 (2.8, 6.825) -> (0.25, 6.825)
  line L666 (0.25, 6.825) -> (0.25, 7.275)
  line L667 (0.25, 6.675) -> (2.8, 6.675)
  line L668 (2.8, 6.675) -> (2.8, 6.225)
  line L669 (2.8, 6.225) -> (0.25, 6.225)
  line L670 (0.25, 6.225) -> (0.25, 6.675)
  line L671 (0.25, 6.075) -> (2.8, 6.075)
  line L672 (2.8, 6.075) -> (2.8, 5.625)
  line L673 (2.8, 5.625) -> (0.25, 5.625)
  line L674 (0.25, 5.625) -> (0.25, 6.075)
  line L675 (0.25, 5.475) -> (2.8, 5.475)
  line L676 (2.8, 5.475) -> (2.8, 5.025)
  line L677 (2.8, 5.025) -> (0.25, 5.025)
  line L678 (0.25, 5.025) -> (0.25, 5.475)
  line L679 (0.25, 4.875) -> (2.8, 4.875)
  line L680 (2.8, 4.875) -> (2.8, 4.425)
  line L681 (2.8, 4.425) -> (0.25, 4.425)
  line L682 (0.25, 4.425) -> (0.25, 4.875)
  line L683 (0.25, 4.275) -> (2.8, 4.275)
  line L684 (2.8, 4.275) -> (2.8, 3.825)
  line L685 (2.8, 3.825) -> (0.25, 3.825)
  line L686 (0.25, 3.825) -> (0.25, 4.275)
  line L687 (0.25, 3.675) -> (2.8, 3.675)
  line L688 (2.8, 3.675) -> (2.8, 3.225)
  line L689 (2.8, 3.225) -> (0.25, 3.225)
  line L690 (0.25, 3.225) -> (0.25, 3.675)
  line L691 (0.25, 3.075) -> (2.8, 3.075)
  line L692 (2.8, 3.075) -> (2.8, 2.625)
  line L693 (2.8, 2.625) -> (0.25, 2.625)
  line L694 (0.25, 2.625) -> (0.25, 3.075)
  line L695 (0.25, 2.475) -> (2.8, 2.475)
  line L696 (2.8, 2.475) -> (2.8, 2.025)
  line L697 (2.8, 2.025) -> (0.25, 2.025)
  line L698 (0.25, 2.025) -> (0.25, 2.475)
  line L699 (0.25, 1.875) -> (2.8, 1.875)
  line L700 (2.8, 1.875) -> (2.8, 1.425)
  line L701 (2.8, 1.425) -> (0.25, 1.425)
  line L702 (0.25, 1.425) -> (0.25, 1.875)
  line L703 (0.25, 1.275) -> (2.8, 1.275)
  line L704 (2.8, 1.275) -> (2.8, 0.825)
  line L705 (2.8, 0.825) -> (0.25, 0.825)
  line L706 (0.25, 0.825) -> (0.25, 1.275)
  line L707 (0.25, 0.675) -> (2.8, 0.675)
  line L708 (2.8, 0.675) -> (2.8, 0.225)
  line L709 (2.8, 0.225) -> (0.25, 0.225)
  line L710 (0.25, 0.225) -> (0.25, 0.675)
  line L711 (0.25, 0.075) -> (2.8, 0.075)
  line L712 (2.8, 0.075) -> (2.8, -0.375)
  line L713 (2.8, -0.375) -> (0.25, -0.375)
  line L714 (0.25, -0.375) -> (0.25, 0.075)
  line L715 (0.25, -0.525) -> (2.8, -0.525)
  line L716 (2.8, -0.525) -> (2.8, -0.975)
  line L717 (2.8, -0.975) -> (0.25, -0.975)
  line L718 (0.25, -0.975) -> (0.25, -0.525)
  line L719 (0.25, -1.125) -> (2.8, -1.125)
  line L720 (2.8, -1.125) -> (2.8, -1.575)
  line L721 (2.8, -1.575) -> (0.25, -1.575)
  line L722 (0.25, -1.575) -> (0.25, -1.125)
  line L723 (0.25, -1.725) -> (2.8, -1.725)
  line L724 (2.8, -1.725) -> (2.8, -2.175)
  line L725 (2.8, -2.175) -> (0.25, -2.175)
  line L726 (0.25, -2.175) -> (0.25, -1.725)
  line L727 (0.25, -2.325) -> (2.8, -2.325)
  line L728 (2.8, -2.325) -> (2.8, -2.775)
  line L729 (2.8, -2.775) -> (0.25, -2.775)
  line L730 (0.25, -2.775) -> (0.25, -2.325)
  line L731 (0.25, -2.925) -> (2.8, -2.925)
  line L732 (2.8, -2.925) -> (2.8, -3.375)
  line L733 (2.8, -3.375) -> (0.25, -3.375)
  line L734 (0.25, -3.375) -> (0.25, -2.925)
  line L735 (0.25, -3.525) -> (2.8, -3.525)
  line L736 (2.8, -3.525) -> (2.8, -3.975)
  line L737 (2.8, -3.975) -> (0.25, -3.975)
  line L738 (0.25, -3.975) -> (0.25, -3.525)
  line L739 (0.25, -4.125) -> (2.8, -4.125)
  line L740 (2.8, -4.125) -> (2.8, -4.575)
  line L741 (2.8, -4.575) -> (0.25, -4.575)
  line L742 (0.25, -4.575) -> (0.25, -4.125)
  line L743 (0.25, -4.725) -> (2.8, -4.725)
  line L744 (2.8, -4.725) -> (2.8, -5.175)
  line L745 (2.8, -5.175) -> (0.25, -5.175)
  line L746 (0.25, -5.175) -> (0.25, -4.725)
  line L747 (0.25, -5.325) -> (2.8, -5.325)
  line L748 (2.8, -5.325) -> (2.8, -5.775)
  line L749 (2.8, -5.775) -> (0.25, -5.775)
  line L750 (0.25, -5.775) -> (0.25, -5.325)
  line L751 (0.25, -5.925) -> (2.8, -5.925)
  line L752 (2.8, -5.925) -> (2.8, -6.375)
  line L753 (2.8, -6.375) -> (0.25, -6.375)
  line L754 (0.25, -6.375) -> (0.25, -5.925)
  line L755 (0.25, -6.525) -> (2.8, -6.525)
  line L756 (2.8, -6.525) -> (2.8, -6.975)
  line L757 (2.8, -6.975) -> (0.25, -6.975)
  line L758 (0.25, -6.975) -> (0.25, -6.525)
  line L759 (0.25, -7.125) -> (2.8, -7.125)
  line L760 (2.8, -7.125) -> (2.8, -7.575)
  line L761 (2.8, -7.575) -> (0.25, -7.575)
  line L762 (0.25, -7.575) -> (0.25, -7.125)
  line L763 (0.25, -7.725) -> (2.8, -7.725)
  line L764 (2.8, -7.725) -> (2.8, -8.175)
  line L765 (2.8, -8.175) -> (0.25, -8.175)
  line L766 (0.25, -8.175) -> (0.25, -7.725)
  line L767 (0.25, -8.325) -> (2.8, -8.325)
  line L768 (2.8, -8.325) -> (2.8, -8.775)
  line L769 (2.8, -8.775) -> (0.25, -8.775)
  line L770 (0.25, -8.775) -> (0.25, -8.325)
  line L771 (0.25, -8.925) -> (2.8, -8.925)
  line L772 (2.8, -8.925) -> (2.8, -9.375)
  line L773 (2.8, -9.375) -> (0.25, -9.375)
  line L774 (0.25, -9.375) -> (0.25, -8.925)
  line L775 (0.25, -9.525) -> (2.8, -9.525)
  line L776 (2.8, -9.525) -> (2.8, -9.975)
  line L777 (2.8, -9.975) -> (0.25, -9.975)
  line L778 (0.25, -9.975) -> (0.25, -9.525)
  line L779 (0.25, -10.125) -> (2.8, -10.125)
  line L780 (2.8, -10.125) -> (2.8, -10.575)
  line L781 (2.8, -10.575) -> (0.25, -10.575)
  line L782 (0.25, -10.575) -> (0.25, -10.125)
  line L783 (0.25, -10.725) -> (2.8, -10.725)
  line L784 (2.8, -10.725) -> (2.8, -11.175)
  line L785 (2.8, -11.175) -> (0.25, -11.175)
  line L786 (0.25, -11.175) -> (0.25, -10.725)
  line L787 (0.25, -11.325) -> (2.8, -11.325)
  line L788 (2.8, -11.325) -> (2.8, -11.775)
  line L789 (2.8, -11.775) -> (0.25, -11.775)
  line L790 (0.25, -11.775) -> (0.25, -11.325)
  line L791 (0.25, -11.925) -> (2.8, -11.925)
  line L792 (2.8, -11.925) -> (2.8, -12.375)
  line L793 (2.8, -12.375) -> (0.25, -12.375)
  line L794 (0.25, -12.375) -> (0.25, -11.925)
  line L795 (0.25, -12.525) -> (2.8, -12.525)
  line L796 (2.8, -12.525) -> (2.8, -12.975)
  line L797 (2.8, -12.975) -> (0.25, -12.975)
  line L798 (0.25, -12.975) -> (0.25, -12.525)
  line L799 (0.25, -13.125) -> (2.8, -13.125)
  line L800 (2.8, -13.125) -> (2.8, -13.575)
  line L801 (2.8, -13.575) -> (0.25, -13.575)
  line L802 (0.25, -13.575) -> (0.25, -13.125)
  line L803 (0.25, -13.725) -> (2.8, -13.725)
  line L804 (2.8, -13.725) -> (2.8, -14.175)
  line L805 (2.8, -14.175) -> (0.25, -14.175)
  line L806 (0.25, -14.175) -> (0.25, -13.725)
  line L807 (0.25, -14.325) -> (2.8, -14.325)
  line L808 (2.8, -14.325) -> (2.8, -14.775)
  line L809 (2.8, -14.775) -> (0.25, -14.775)
  line L810 (0.25, -14.775) -> (0.25, -14.325)
  line L811 (0.25, -14.925) -> (2.8, -14.925)
  line L812 (2.8, -14.925) -> (2.8, -15.375)
  line L813 (2.8, -15.375) -> (0.25, -15.375)
  line L814 (0.25, -15.375) -> (0.25, -14.925)
  line L815 (0.25, -15.525) -> (2.8, -15.525)
  line L816 (2.8, -15.525) -> (2.8, -15.975)
  line L817 (2.8, -15.975) -> (0.25, -15.975)
  line L818 (0.25, -15.975) -> (0.25, -15.525)
  line L819 (0.25, -16.125) -> (2.8, -16.125)
  line L820 (2.8, -16.125) -> (2.8, -16.575)
  line L821 (2.8, -16.575) -> (0.25, -16.575)
  line L822 (0.25, -16.575) -> (0.25, -16.125)
  line L823 (0.25, -16.725) -> (2.8, -16.725)
  line L824 (2.8, -16.725) -> (2.8, -17.175)
  line L825 (2.8, -17.175) -> (0.25, -17.175)
  line L826 (0.25, -17.175) -> (0.25, -16.725)
  line L827 (0.25, -17.325) -> (2.8, -17.325)
  line L828 (2.8, -17.325) -> (2.8, -17.775)
  line L829 (2.8, -17.775) -> (0.25, -17.775)
  line L830 (0.25, -17.775) -> (0.25, -17.325)
  line L831 (0.25, -17.925) -> (2.8, -17.925)
  line L832 (2.8, -17.925) -> (2.8, -18.375)
  line L833 (2.8, -18.375) -> (0.25, -18.375)
  line L834 (0.25, -18.375) -> (0.25, -17.925)
  line L835 (0.25, -18.525) -> (2.8, -18.525)
  line L836 (2.8, -18.525) -> (2.8, -18.975)
  line L837 (2.8, -18.975) -> (0.25, -18.975)
  line L838 (0.25, -18.975) -> (0.25, -18.525)
  line L839 (0.25, -19.125) -> (2.8, -19.125)
  line L840 (2.8, -19.125) -> (2.8, -19.575)
  line L841 (2.8, -19.575) -> (0.25, -19.575)
  line L842 (0.25, -19.575) -> (0.25, -19.125)
  line L843 (0.25, -19.725) -> (2.8, -19.725)
  line L844 (2.8, -19.725) -> (2.8, -20.175)
  line L845 (2.8, -20.175) -> (0.25, -20.175)
  line L846 (0.25, -20.175) -> (0.25, -19.725)
  line L847 (0.25, -20.325) -> (2.8, -20.325)
  line L848 (2.8, -20.325) -> (2.8, -20.775)
  line L849 (2.8, -20.775) -> (0.25, -20.775)
  line L850 (0.25, -20.775) -> (0.25, -20.325)
  line L851 (0.25, -20.925) -> (2.8, -20.925)
  line L852 (2.8, -20.925) -> (2.8, -21.375)
  line L853 (2.8, -21.375) -> (0.25, -21.375)
  line L854 (0.25, -21.375) -> (0.25, -20.925)
  line L855 (0.25, -21.525) -> (2.8, -21.525)
  line L856 (2.8, -21.525) -> (2.8, -21.975)
  line L857 (2.8, -21.975) -> (0.25, -21.975)
  line L858 (0.25, -21.975) -> (0.25, -21.525)
  line L859 (0.25, -22.125) -> (2.8, -22.125)
  line L860 (2.8, -22.125) -> (2.8, -22.575)
  line L861 (2.8, -22.575) -> (0.25, -22.575)
  line L862 (0.25, -22.575) -> (0.25, -22.125)
  line L863 (0.25, -22.725) -> (2.8, -22.725)
  line L864 (2.8, -22.725) -> (2.8, -23.175)
  line L865 (2.8, -23.175) -> (0.25, -23.175)
  line L866 (0.25, -23.175) -> (0.25, -22.725)
  line L867 (0.25, -23.325) -> (2.8, -23.325)
  line L868 (2.8, -23.325) -> (2.8, -23.775)
  line L869 (2.8, -23.775) -> (0.25, -23.775)
  line L870 (0.25, -23.775) -> (0.25, -23.325)
  line L871 (0.25, -23.925) -> (2.8, -23.925)
  line L872 (2.8, -23.925) -> (2.8, -24.375)
  line L873 (2.8, -24.375) -> (0.25, -24.375)
  line L874 (0.25, -24.375) -> (0.25, -23.925)
  line L875 (0.25, -24.525) -> (2.8, -24.525)
  line L876 (2.8, -24.525) -> (2.8, -24.975)
  line L877 (2.8, -24.975) -> (0.25, -24.975)
  line L878 (0.25, -24.975) -> (0.25, -24.525)
  line L879 (0.25, -25.125) -> (2.8, -25.125)
  line L880 (2.8, -25.125) -> (2.8, -25.575)
  line L881 (2.8, -25.575) -> (0.25, -25.575)
  line L882 (0.25, -25.575) -> (0.25, -25.125)
  line L883 (0.25, -25.725) -> (2.8, -25.725)
  line L884 (2.8, -25.725) -> (2.8, -26.175)
  line L885 (2.8, -26.175) -> (0.25, -26.175)
  line L886 (0.25, -26.175) -> (0.25, -25.725)
  line L887 (0.25, -26.325) -> (2.8, -26.325)
  line L888 (2.8, -26.325) -> (2.8, -26.775)
  line L889 (2.8, -26.775) -> (0.25, -26.775)
  line L890 (0.25, -26.775) -> (0.25, -26.325)
  line L891 (0.25, -26.925) -> (2.8, -26.925)
  line L892 (2.8, -26.925) -> (2.8, -27.375)
  line L893 (2.8, -27.375) -> (0.25, -27.375)
  line L894 (0.25, -27.375) -> (0.25, -26.925)
  line L895 (0.25, -27.525) -> (2.8, -27.525)
  line L896 (2.8, -27.525) -> (2.8, -27.975)
  line L897 (2.8, -27.975) -> (0.25, -27.975)
  line L898 (0.25, -27.975) -> (0.25, -27.525)
  line L899 (0.25, -28.125) -> (2.8, -28.125)
  line L900 (2.8, -28.125) -> (2.8, -28.575)
  line L901 (2.8, -28.575) -> (0.25, -28.575)
  line L902 (0.25, -28.575) -> (0.25, -28.125)
  line L903 (0.25, -28.725) -> (2.8, -28.725)
  line L904 (2.8, -28.725) -> (2.8, -29.175)
  line L905 (2.8, -29.175) -> (0.25, -29.175)
  line L906 (0.25, -29.175) -> (0.25, -28.725)
  line L907 (0.25, -29.325) -> (2.8, -29.325)
  line L908 (2.8, -29.325) -> (2.8, -29.775)
  line L909 (2.8, -29.775) -> (0.25, -29.775)
  line L910 (0.25, -29.775) -> (0.25, -29.325)
  line L911 (0.25, -29.925) -> (2.8, -29.925)
  line L912 (2.8, -29.925) -> (2.8, -30.375)
  line L913 (2.8, -30.375) -> (0.25, -30.375)
  line L914 (0.25, -30.375) -> (0.25, -29.925)
  line L915 (0.25, -30.525) -> (2.8, -30.525)
  line L916 (2.8, -30.525) -> (2.8, -30.975)
  line L917 (2.8, -30.975) -> (0.25, -30.975)
  line L918 (0.25, -30.975) -> (0.25, -30.525)
  line L919 (0.25, -31.125) -> (2.8, -31.125)
  line L920 (2.8, -31.125) -> (2.8, -31.575)
  line L921 (2.8, -31.575) -> (0.25, -31.575)
  line L922 (0.25, -31.575) -> (0.25, -31.125)
  point P0 (0, 0)
  point P1 (0.25, 16.05)
  point P2 (0.25, 20.25)
  dimension "d101" = 0.25
  dimension "d102" = 2.55
  dimension "d103" = 0.45
  dimension "d107" = 0.6
  dimension "d114" = 0.6
  dimension "d119" = 4.2
  dimension "d120" = 1.8
  constraints: 800 end point, 4 parallel, 3 collinear, 2 horizontal, 2 midpoint, 2 perpendicular, 2 vertical, 784 other
  measures "d101" distance between parallel lines of L526 L522
  measures "d102" distance of L523.start L523.end
  measures "d103" distance of L525.end L523.start
  measures "d107" distance of L523.end L531.start
  measures "d114" distance of L527.start L607.start
  measures "d119" distance of point (0.25, 20.25) point (0.25, 16.05)
  measures "d120" vertical distance of point (0.25, 20.25) A0.centre
extrude "Extrusion7" add sketch "Sketch7" along normal blind 0.035 contours L523 L524 L525 L526 | L527 L528 L529 L530 | L531 L533 L532 L534 | L535 L537 L536 L538 | L539 L541 L540 L542 | L543 L545 L544 L546 | L547 L549 L548 L550 | L551 L553 L552 L554 | L555 L557 L556 L558 | L559 L561 L560 L562 | L563 L565 L564 L566 | L567 L569 L568 L570 | L571 L573 L572 L574 | L575 L577 L576 L578 | L579 L581 L580 L582 | L583 L585 L584 L586 | L587 L589 L588 L590 | L591 L593 L592 L594 | L595 L597 L596 L598 | L599 L601 L600 L602 | L603 L605 L604 L606 | L607 L608 L609 L610 | L611 L612 L613 L614 | L615 L616 L617 L618 | L619 L620 L621 L622 | L623 L624 L625 L626 | L627 L628 L629 L630 | L631 L632 L633 L634 | L635 L636 L637 L638 | L639 L640 L641 L642 | L643 L644 L645 L646 | L647 L648 L649 L650 | L651 L652 L653 L654 | L655 L656 L657 L658 | L659 L660 L661 L662 | L663 L664 L665 L666 | L667 L668 L669 L670 | L671 L672 L673 L674 | L675 L676 L677 L678 | L679 L680 L681 L682 | L683 L684 L685 L686 | L687 L688 L689 L690 | L691 L692 L693 L694 | L695 L696 L697 L698 | L699 L700 L701 L702 | L703 L704 L705 L706 | L707 L708 L709 L710 | L711 L712 L713 L714 | L715 L716 L717 L718 | L719 L720 L721 L722 | L723 L724 L725 L726 | L727 L728 L729 L730 | L731 L732 L733 L734 | L735 L736 L737 L738 | L739 L740 L741 L742 | L743 L744 L745 L746 | L747 L748 L749 L750 | L751 L752 L753 L754 | L755 L756 L757 L758 | L759 L760 L761 L762 | L763 L764 L765 L766 | L767 L768 L769 L770 | L771 L772 L773 L774 | L775 L776 L777 L778 | L779 L780 L781 L782 | L783 L784 L785 L786 | L787 L788 L789 L790 | L791 L792 L793 L794 | L795 L796 L797 L798 | L799 L800 L801 L802 | L803 L804 L805 L806 | L807 L808 L809 L810 | L811 L812 L813 L814 | L815 L816 L817 L818 | L819 L820 L821 L822 | L823 L824 L825 L826 | L827 L828 L829 L830 | L831 L832 L833 L834 | L835 L836 L837 L838 | L839 L840 L841 L842 | L843 L844 L845 L846 | L847 L848 L849 L850 | L851 L852 L853 L854 | L855 L856 L857 L858 | L859 L860 L861 L862 | L863 L864 L865 L866 | L867 L868 L869 L870 | L871 L872 L873 L874 | L875 L876 L877 L878 | L879 L880 L881 L882 | L883 L884 L885 L886 | L887 L888 L889 L890 | L891 L892 L893 L894 | L895 L896 L897 L898 | L899 L900 L901 L902 | L903 L904 L905 L906 | L907 L908 L909 L910 | L911 L912 L913 L914 | L915 L916 L917 L918 | L919 L920 L921 L922
fillet "Fillet1" radius 1 8 edges at (12.5, 47.9, 0) (0, 33.8, 0) (12.5, 33.8, 0) (0, -33.8, 0) (12.5, -33.8, 0) (12.5, -47.9, 0) (91.4, -47.9, 0) (91.4, 47.9, 0)